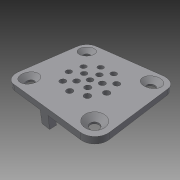
# Autodesk Inventor part: dht22_case_top
Saved by Autodesk Inventor 2014 (Build 180170000, 170)
## iProperties
Created: 2016-01-31
Part Number: dht22_case_top
Material: Generic
Document SubType Name: Modeling
Designer: buben
Density: 1 g/cm^3
Appearance: Default
Author: buben
Autodesk Inventor part; units mm, degrees
ref_plane "YZ Plane" through (0, 0, 0) normal (1, 0, 0) x (0, 1, 0)
ref_plane "XZ Plane" through (0, 0, 0) normal (0, 1, 0) x (-1, 0, 0)
ref_plane "XY Plane" through (0, 0, 0) normal (0, 0, 1) x (1, 0, 0)
sketch "Sketch1" plane through (0, 0, 0) normal (0, 1, 0) x (-1, 0, 0)
  line L0 (0, 0) -> (-47, 0)
  line L1 (-47, 0) -> (-47, -43)
  line L2 (-47, -43) -> (0, -43)
  line L3 (0, -43) -> (0, 0)
  dimension "d0" = 43
  dimension "d1" = 47
  constraints: 8 end point, 2 parallel, 1 horizontal, 1 perpendicular
  measures "d0" distance of L2.end L0.start
  measures "d1" distance of L0.start L0.end
extrude "Extrusion1" add sketch "Sketch1" along normal blind 3
sketch "Sketch2" plane through (0, 3, 0) normal (0, 1, 0) x (1, 0, 0)
  line L0 (47, 43) -> (0, 43) projected
  line L1 (0, 43) -> (0, 0) projected
  line L2 (6.5, 36.5) -> (40.5, 36.5) construction
  line L3 (40.5, 36.5) -> (40.5, 6.5) construction
  line L4 (40.5, 6.5) -> (6.5, 6.5) construction
  line L5 (6.5, 6.5) -> (6.5, 36.5) construction
  point P0 (23.5, 36.5)
  point P1 (23.5, 43)
  point P2 (6.5, 21.5)
  point P3 (0, 21.5)
  dimension "d4" = 6.5
  dimension "d5" = 6.5
  constraints: 8 end point, 4 coincident, 4 midpoint, 2 parallel, 1 horizontal, 1 horizontal alignment, 1 perpendicular, 1 vertical alignment
  measures "d4" distance from line of L1 point (6.5, 6.5)
  measures "d5" distance between parallel lines of L0 L2
hole "Hole1" at (6.5, 3, -6.5) at (6.5, 3, -36.5) at (40.5, 3, -36.5) at (40.5, 3, -6.5) direction (0, -1, 0) diameter 4 end through all countersink diameter 8.5 countersink angle 90
sketch "Sketch3" plane through (0, 0, 0) normal (0, -1, 0) x (1, 0, 0)
  line L0 (0, 0) -> (47, 0) projected
  line L1 (21.4, 0) -> (25.6, 0)
  line L2 (25.6, 0) -> (25.6, -3)
  line L3 (25.6, -3) -> (21.4, -3)
  line L4 (21.4, -3) -> (21.4, 0)
  point P0 (23.5, -3)
  point P1 (23.5, 0)
  dimension "d13" = 4.2
  dimension "d14" = 3
  constraints: 8 end point, 2 midpoint, 2 parallel, 1 horizontal, 1 perpendicular, 1 point on line, 1 vertical alignment
  measures "d13" distance of L2.end L3.end
  measures "d14" distance of L1.end L2.end
extrude "Extrusion2" add sketch "Sketch3" along normal blind 6.2
sketch "Sketch4" plane through (0, 3, 0) normal (0, 1, 0) x (1, 0, 0)
  line L0 (47, 43) -> (0, 43) projected
  line L1 (0, 43) -> (0, 0) projected
  circle A0 centre (23.5, 21.5) radius 1.5
  circle A1 centre (23.5, 26.5) radius 1.5
  circle A2 centre (18.7447, 23.0451) radius 1.5
  circle A3 centre (20.5611, 17.4549) radius 1.5
  circle A4 centre (26.4389, 17.4549) radius 1.5
  circle A5 centre (28.2553, 23.0451) radius 1.5
  circle A6 centre (23.5, 11.5) radius 1.5
  circle A7 centre (29.9279, 13.8396) radius 1.5
  circle A8 centre (33.3481, 19.7635) radius 1.5
  circle A9 centre (32.1603, 26.5) radius 1.5
  circle A10 centre (26.9202, 30.8969) radius 1.5
  circle A11 centre (20.0798, 30.8969) radius 1.5
  circle A12 centre (14.8397, 26.5) radius 1.5
  circle A13 centre (13.6519, 19.7635) radius 1.5
  circle A14 centre (17.0721, 13.8396) radius 1.5
  point P0 (23.5, 43)
  point P1 (0, 21.5)
  dimension "d17" = 3
  dimension "d18" = 3
  dimension "d19" = 5
  dimension "d22" = 360
  dimension "d24" = 3
  dimension "d25" = 10
  dimension "d28" = 360
  constraints: 15 centre point, 3 vertical alignment, 2 midpoint, 1 coincident, 1 horizontal alignment, 30 other
  measures "d17" diameter of A0
  measures "d18" diameter of A1
  measures "d19" distance of A1.centre point (23.5, 21.5)
  measures "d24" diameter of A6
  measures "d25" distance of A0.centre A6.centre
extrude "Extrusion3" cut sketch "Sketch4" against normal through all
fillet "Fillet1" radius 6 4 edges at (0, 1.5, -43) (0, 1.5, 0) (47, 1.5, 0) (47, 1.5, -43)
equation "\"d5\" = d4"
equation "\"d18\" = d17"
equation "\"d24\" = d17"
body "Solid1"
